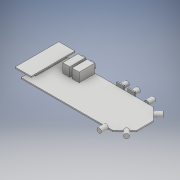
# Autodesk Inventor part: ADF4355-2_EVB
Saved by Autodesk Inventor 2018 (Build 220112000, 112)
## iProperties
Created: 2018-01-02
Part Number: ADF4355-2_EVB
Material: Generic
Document SubType Name: Modeling
Designer: rwradema
Density: 1 g/cm^3
Appearance: Default
Author: rwradema
Autodesk Inventor part; units mm, degrees
ref_plane "YZ Plane" through (0, 0, 0) normal (1, 0, 0) x (0, 1, 0)
ref_plane "XZ Plane" through (0, 0, 0) normal (0, 1, 0) x (-1, 0, 0)
ref_plane "XY Plane" through (0, 0, 0) normal (0, 0, 1) x (1, 0, 0)
sketch "Sketch1" plane through (0, 0, 0) normal (0, 0, 1) x (1, 0, 0)
  line L0 (-60.6356, 29.0823) -> (-60.6356, -26.6177)
  line L1 (-60.6356, -26.6177) -> (64.8902, -26.6177)
  line L2 (64.8902, -26.6177) -> (81.3644, -10.5677)
  line L3 (81.3644, -10.5677) -> (81.3644, 13.0323)
  line L4 (81.3644, 13.0323) -> (64.8902, 29.0823)
  line L5 (64.8902, 29.0823) -> (-60.6356, 29.0823)
  line L6 (-97.195, 1.2323) -> (98.286, 1.2323) construction
  point P0 (0, 0)
  dimension "d2" = 142
  dimension "d3" = 55.7
  dimension "d4" = 23.6
  dimension "d5" = 23
  constraints: 14 end point, 3 parallel, 1 horizontal, 1 perpendicular, 1 vertical, 1 other
  measures "d2" distance between parallel lines of L0 L3
  measures "d3" distance of L0.start L0.end
  measures "d4" distance of L2.end L3.end
  measures "d5" distance of L3.end L4.end
extrude "Extrusion1" add sketch "Sketch1" along normal blind 1.6
sketch "Sketch2" plane through (0, 0, 1.6) normal (0, 0, 1) x (1, 0, 0)
  line L0 (39.3644, 30.5823) -> (29.7644, 30.5823)
  line L1 (29.7644, 30.5823) -> (29.7644, 29.0823)
  line L2 (29.7644, 29.0823) -> (39.3644, 29.0823)
  line L3 (39.3644, 29.0823) -> (39.3644, 30.5823)
  line L4 (39.3644, 30.5823) -> (29.7644, 29.0823) construction
  line L5 (29.7644, 30.5823) -> (39.3644, 29.0823) construction
  line L6 (24.2144, 30.5823) -> (14.6144, 30.5823)
  line L7 (14.6144, 30.5823) -> (14.6144, 29.0823)
  line L8 (14.6144, 29.0823) -> (24.2144, 29.0823)
  line L9 (24.2144, 29.0823) -> (24.2144, 30.5823)
  line L10 (24.2144, 30.5823) -> (14.6144, 29.0823) construction
  line L11 (14.6144, 30.5823) -> (24.2144, 29.0823) construction
  line L12 (64.8902, 29.0823) -> (-60.6356, 29.0823) projected
  line L13 (-60.6356, 29.0823) -> (-60.6356, -26.6177) projected
  point P0 (0, 0)
  point P1 (34.5644, 29.8323)
  point P2 (19.4144, 29.8323)
  dimension "d6" = 9.6
  dimension "d7" = 1.5
  dimension "d8" = 84.85
  dimension "d9" = 100
  constraints: 24 end point, 4 midpoint, 4 parallel, 2 equal length, 2 horizontal, 2 perpendicular, 1 collinear, 1 point on line
  measures "d6" distance of L6.start L6.end
  measures "d7" distance of L6.end L7.end
  measures "d8" distance between parallel lines of L13 L9
  measures "d9" distance between parallel lines of L13 L3
extrude "Extrusion2" add sketch "Sketch2" along normal blind 4.4
sketch "Sketch3" plane through (0, 0, 1.6) normal (0, 0, -1) x (-1, 0, 0)
  line L0 (-39.3644, 30.5823) -> (-29.7644, 30.5823) projected
  line L1 (-29.7644, 29.0823) -> (-24.2144, 29.0823) projected
  line L2 (-39.3644, 30.5823) -> (-29.7644, 30.5823)
  line L3 (-29.7644, 30.5823) -> (-29.7644, 29.0823)
  line L4 (-29.7644, 29.0823) -> (-39.3644, 29.0823)
  line L5 (-39.3644, 29.0823) -> (-39.3644, 30.5823)
  line L6 (-24.2144, 30.5823) -> (-14.6144, 30.5823) projected
  line L7 (-24.2144, 30.5823) -> (-14.6144, 30.5823)
  line L8 (-14.6144, 30.5823) -> (-14.6144, 29.0823)
  line L9 (-14.6144, 29.0823) -> (-24.2144, 29.0823)
  line L10 (-24.2144, 29.0823) -> (-24.2144, 30.5823)
  point P0 (0, 0)
  constraints: 16 end point, 4 parallel, 2 horizontal, 2 perpendicular, 1 point on line
extrude "Extrusion3" add sketch "Sketch3" along normal blind 3.67
sketch "Sketch4" plane through (14.6144, 30.5823, 6) normal (0, 1, 0) x (1, 0, 0)
  line L0 (0, 0) -> (9.6, 0) construction
  line L1 (4.8, 0) -> (4.8, 8.07) construction
  line L2 (9.6, 8.07) -> (0, 8.07) construction
  circle A0 centre (4.8, 4.035) radius 3.115
  line L3 (15.15, 0) -> (24.75, 0) construction
  line L4 (19.95, 0) -> (19.95, 8.07) construction
  line L5 (24.75, 8.07) -> (15.15, 8.07) construction
  circle A1 centre (19.95, 4.035) radius 3.115
  point P0 (-14.6144, 6)
  dimension "d14" = 6.23
  constraints: 6 midpoint, 4 end point, 2 centre point, 1 equal radius
  measures "d14" diameter of A0
extrude "Extrusion4" add sketch "Sketch4" along normal blind 8
sketch "Sketch5" plane through (64.8902, 29.0823, 1.6) normal (0.6978261, 0.7162672, 0) x (0.7162672, -0.6978261, 0)
  line L0 (23, 0) -> (0, 0) projected
  circle A0 centre (12.6, 0) radius 3.11
  point P0 (-26.1844, 1.6)
  dimension "d17" = 12.6
  dimension "d18" = 6.22
  constraints: 1 centre point, 1 point on line
  measures "d17" distance of A0.centre L0.end
  measures "d18" diameter of A0
extrude "Extrusion5" add sketch "Sketch5" along normal blind 9.5
sketch "Sketch6" plane through (81.3644, -10.5677, 0) normal (0.6978261, -0.7162672, 0) x (0.7162672, 0.6978261, 0)
  line L0 (-20.142, 1.6) -> (-74.0411, 1.6) projected
  circle A0 centre (-9.5, 1.6) radius 3.1
  line L1 (-23, 0) -> (-23, 1.6) projected
  line L2 (0, 0) -> (0, 1.6) projected
  point P0 (-50.9042, 0)
  dimension "d22" = 6.2
  dimension "d25" = 9.5
  constraints: 1 centre point, 1 point on line
  measures "d22" diameter of A0
  measures "d25" distance from line of L2 A0.centre
extrude "Extrusion6" add sketch "Sketch6" along normal blind 9.5
sketch "Sketch7" plane through (-60.6356, -26.6177, 0) normal (0, -1, 0) x (1, 0, 0)
  line L0 (125.5259, 1.6) -> (100, 1.6) projected
  circle A0 centre (116.5259, 1.6) radius 3.125
  point P0 (60.6356, 0)
  dimension "d26" = 9
  dimension "d27" = 6.25
  constraints: 1 centre point, 1 point on line
  measures "d26" distance of A0.centre L0.start
  measures "d27" diameter of A0
extrude "Extrusion7" add sketch "Sketch7" along normal blind 9.5
sketch "Sketch8" plane through (64.8902, 29.0823, 1.6) normal (0, 1, 0) x (1, 0, 0)
  line L0 (0, 0) -> (-25.5259, 0) projected
  circle A0 centre (-9, 0) radius 3.125
  point P0 (-64.8902, 1.6)
  dimension "d30" = 6.25
  dimension "d31" = 9
  constraints: 1 centre point, 1 point on line
  measures "d30" diameter of A0
  measures "d31" distance of L0.start A0.centre
extrude "Extrusion8" add sketch "Sketch8" along normal blind 9.5
sketch "Sketch9" plane through (0, 0, 1.6) normal (0, 0, 1) x (1, 0, 0)
  line L0 (-37.1356, 27.8723) -> (-27.3856, 27.8723)
  line L1 (-27.3856, 27.8723) -> (-27.3856, 6.8723)
  line L2 (-27.3856, 6.8723) -> (-37.1356, 6.8723)
  line L3 (-37.1356, 6.8723) -> (-37.1356, 27.8723)
  line L4 (-37.1356, 27.8723) -> (-27.3856, 6.8723) construction
  line L5 (-27.3856, 27.8723) -> (-37.1356, 6.8723) construction
  line L6 (-24.3856, 27.8723) -> (-14.6356, 27.8723)
  line L7 (-14.6356, 27.8723) -> (-14.6356, 6.8723)
  line L8 (-14.6356, 6.8723) -> (-24.3856, 6.8723)
  line L9 (-24.3856, 6.8723) -> (-24.3856, 27.8723)
  line L10 (-24.3856, 27.8723) -> (-14.6356, 6.8723) construction
  line L11 (-14.6356, 27.8723) -> (-24.3856, 6.8723) construction
  line L12 (14.6144, 29.0823) -> (-60.6356, 29.0823) projected
  line L13 (-60.6356, 29.0823) -> (-60.6356, -26.6177) projected
  point P0 (0, 0)
  point P1 (-32.2606, 17.3723)
  point P2 (-19.5106, 17.3723)
  dimension "d34" = 9.75
  dimension "d35" = 21
  dimension "d36" = 1.21
  dimension "d37" = 23.5
  dimension "d38" = 36.25
  constraints: 24 end point, 4 midpoint, 4 parallel, 2 equal length, 2 horizontal, 2 perpendicular, 1 point on line
  measures "d34" distance of L6.start L6.end
  measures "d35" distance of L6.end L7.end
  measures "d36" distance between parallel lines of L12 L6
  measures "d37" distance between parallel lines of L13 L3
  measures "d38" distance between parallel lines of L13 L9
extrude "Extrusion9" add sketch "Sketch9" along normal blind 12.6
sketch "Sketch10" plane through (-24.3856, 27.8723, 1.6) normal (0, 1, 0) x (1, 0, 0)
  circle A0 centre (-7.875, -7) radius 4.45
  circle A1 centre (4.875, -7) radius 4.45
  line L0 (9.75, -12.6) -> (0, -12.6) projected
  line L1 (-3, -12.6) -> (-12.75, -12.6) projected
  point P0 (24.3856, 1.6)
  dimension "d41" = 5.6
  dimension "d42" = 5.6
  dimension "d43" = 8.9
  constraints: 2 centre point, 1 equal radius
  measures "d41" distance from line of A1.centre L0
  measures "d42" distance from line of L1 A0.centre
  measures "d43" diameter of A0
extrude "Extrusion10" add sketch "Sketch10" along normal blind 2.54
sketch "Sketch11" plane through (0, 0, 1.6) normal (0, 0, 1) x (1, 0, 0)
  line L0 (-57.8356, 27.3823) -> (-52.2356, 27.3823)
  line L1 (-52.2356, 27.3823) -> (-52.2356, -15.2177)
  line L2 (-52.2356, -15.2177) -> (-57.8356, -15.2177)
  line L3 (-57.8356, -15.2177) -> (-57.8356, 27.3823)
  line L4 (-57.8356, 27.3823) -> (-52.2356, -15.2177) construction
  line L5 (-52.2356, 27.3823) -> (-57.8356, -15.2177) construction
  line L6 (14.6144, 29.0823) -> (-60.6356, 29.0823) projected
  line L7 (-60.6356, 29.0823) -> (-60.6356, -26.6177) projected
  point P0 (0, 0)
  point P1 (-55.0356, 6.0823)
  dimension "d46" = 5.6
  dimension "d47" = 42.6
  dimension "d48" = 1.7
  dimension "d49" = 2.8
  constraints: 12 end point, 2 midpoint, 2 parallel, 1 horizontal, 1 perpendicular
  measures "d46" distance of L0.start L0.end
  measures "d47" distance of L2.end L0.start
  measures "d48" distance between parallel lines of L0 L6
  measures "d49" distance between parallel lines of L7 L3
extrude "Extrusion11" add sketch "Sketch11" along normal blind 4.15
sketch "Sketch12" plane through (0, 0, 5.75) normal (0, 0, 1) x (1, 0, 0)
  line L0 (-49.4856, 35.9823) -> (-71.5856, 35.9823)
  line L1 (-71.5856, 35.9823) -> (-71.5856, -24.0177)
  line L2 (-71.5856, -24.0177) -> (-49.4856, -24.0177)
  line L3 (-49.4856, -24.0177) -> (-49.4856, 35.9823)
  line L4 (-52.2356, 27.3823) -> (-57.8356, 27.3823) projected
  line L5 (-57.8356, 27.3823) -> (-57.8356, -15.2177) projected
  point P0 (0, 0)
  dimension "d52" = 22.1
  dimension "d53" = 60
  dimension "d54" = 8.6
  dimension "d55" = 13.75
  constraints: 8 end point, 2 parallel, 1 horizontal, 1 perpendicular
  measures "d52" distance of L0.start L0.end
  measures "d53" distance of L0.end L1.end
  measures "d54" distance between parallel lines of L4 L0
  measures "d55" distance between parallel lines of L1 L5
extrude "Extrusion12" add sketch "Sketch12" along normal blind 1.55
body "Solid1"
